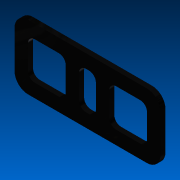
# Autodesk Inventor part: ROV-Side Panel
Saved by Autodesk Inventor 2013 (Build 170138000, 138)
## iProperties
Created: 2014-11-05
Part Number: ROV-Side Panel
Material: Acetal Resin, Black
Document SubType Name: Modeling
Designer: Jeramy
Density: 1 g/cm^3
Author: Jeramy
Autodesk Inventor part; units mm, degrees
ref_plane "YZ Plane" through (0, 0, 0) normal (1, 0, 0) x (0, 1, 0)
ref_plane "XZ Plane" through (0, 0, 0) normal (0, 1, 0) x (-1, 0, 0)
ref_plane "XY Plane" through (0, 0, 0) normal (0, 0, 1) x (1, 0, 0)
sketch "Sketch2" plane through (0, 0, 0) normal (0, 0, 1) x (1, 0, 0)
  line L0 (0, 0) -> (552.641777, 0)
  line L1 (552.641777, 0) -> (552.641777, 244.475)
  line L2 (552.641777, 244.475) -> (0, 244.475)
  line L3 (0, 244.475) -> (0, 0)
  dimension "d6" = 244.475
  constraints: 8 end point, 2 parallel, 1 horizontal, 1 perpendicular
  measures "d6" distance of L1.end L0.end
extrude "Extrusion1" add sketch "Sketch2" along normal blind 19.05
sketch "Sketch3" plane through (0, 0, 19.05) normal (0, 0, 1) x (1, 0, 0)
  line L0 (0, 0) -> (552.641777, 0)
  line L1 (552.641777, 0) -> (552.641777, 244.475)
  line L2 (552.641777, 244.475) -> (0, 244.475)
  line L3 (0, 244.475) -> (0, 0)
  arc A0 (50.896482, 244.475) -> (0, 193.636302) centre (50.799985, 193.675092) ccw
  dimension "d9" = 50.8
  constraints: 2 point on circle, 2 point on line, 1 centre point
  measures "d9" radius of A0
sketch "Sketch3 outline for Extrusion2" plane through (0, 0, 19.05) normal (0, 0, 1) x (1, 0, 0)
  arc A0 (50.896482, 244.475) -> (0, 193.636302) centre (50.799985, 193.675092) ccw
  line L0 (0, 244.475) -> (0, 193.636302)
  line L1 (50.896482, 244.475) -> (0, 244.475)
extrude "Extrusion2" cut sketch "Sketch3 outline for Extrusion2" against normal blind 19.05
sketch "Sketch4" plane through (0, 0, 19.05) normal (0, 0, 1) x (1, 0, 0)
  line L0 (0, 193.713882) -> (0, 0)
  line L1 (0, 0) -> (552.641777, 0)
  line L2 (552.641777, 0) -> (552.641777, 244.475)
  line L3 (552.641777, 244.475) -> (50.703488, 244.475)
  arc A0 (552.641777, 193.713882) -> (500.210663, 244.475) centre (501.841779, 193.701193) ccw
  arc A1 (501.841779, 0) -> (552.641777, 50.788429) centre (501.841778, 50.8) ccw
  arc A2 (0, 50.788429) -> (50.703488, 0) centre (50.799999, 50.799908) ccw
  dimension "d15" = 50.8
  dimension "d16" = 50.8
  dimension "d17" = 50.8
  constraints: 6 point on circle, 6 point on line, 3 centre point
  measures "d15" radius of A0
  measures "d16" radius of A1
  measures "d17" radius of A2
extrude "Extrusion3" cut sketch "Sketch4" against normal blind 19.05 contours A2 L1 L0
sketch "Sketch5" plane through (0, 0, 19.05) normal (0, 0, 1) x (1, 0, 0)
  line L0 (552.641777, 0) -> (552.641777, 244.475)
  line L1 (552.641777, 244.475) -> (50.703488, 244.475)
  arc A0 (552.641777, 193.713882) -> (501.92669, 244.475) centre (501.841792, 193.675071) ccw
  point P0 (0, 0)
  dimension "d20" = 50.8
  constraints: 2 point on circle, 2 point on line, 1 centre point
  measures "d20" radius of A0
extrude "Extrusion4" cut sketch "Sketch5" against normal blind 19.05
sketch "Sketch6" plane through (0, 0, 19.05) normal (0, 0, 1) x (1, 0, 0)
  line L0 (50.703488, 0) -> (552.641777, 0)
  line L1 (552.641777, 0) -> (552.641777, 193.713882)
  arc A0 (501.92669, 0) -> (552.641777, 50.799908) centre (501.841777, 50.799929) ccw
  point P0 (0, 0)
  dimension "d23" = 50.8
  constraints: 2 point on circle, 2 point on line, 1 centre point
  measures "d23" radius of A0
extrude "Extrusion5" cut sketch "Sketch6" against normal blind 19.05
sketch "Sketch7" plane through (0, 0, 19.05) normal (0, 0, 1) x (1, 0, 0)
  arc A0 (552.641777, 193.713882) -> (501.92669, 244.475) centre (501.841792, 193.675071) ccw
  arc A1 (50.703488, 244.475) -> (0, 193.713882) centre (50.799985, 193.675092) ccw
  line L0 (50.799985, 193.675092) -> (193.674985, 193.675092)
  line L1 (193.674985, 193.675092) -> (193.674985, 50.799908)
  line L2 (193.674985, 50.799908) -> (50.799985, 50.799908)
  line L3 (50.799985, 50.799908) -> (50.799985, 193.675092)
  line L4 (501.841792, 193.675071) -> (358.966792, 193.675071)
  line L5 (358.966792, 193.675071) -> (358.966792, 50.799908)
  line L6 (358.966792, 50.799908) -> (501.841792, 50.799908)
  line L7 (501.841792, 50.799908) -> (501.841792, 193.675071)
  point P0 (0, 0)
  dimension "d26" = 142.875
  dimension "d27" = 142.875
  constraints: 16 end point, 4 parallel, 2 horizontal, 2 perpendicular
  measures "d26" distance of L1.end L2.end
  measures "d27" distance of L6.end L5.end
extrude "Extrusion6" cut sketch "Sketch7" against normal blind 19.05 contours L0 L1 L2 L3
sketch "Sketch8" plane through (0, 0, 19.05) normal (0, 0, 1) x (1, 0, 0)
  arc A0 (552.641777, 193.713882) -> (501.92669, 244.475) centre (501.841792, 193.675071) ccw
  line L0 (501.841792, 193.675071) -> (358.966792, 193.675071)
  line L1 (358.966792, 193.675071) -> (358.966792, 50.799908)
  line L2 (358.966792, 50.799908) -> (501.841792, 50.799908)
  line L3 (501.841792, 50.799908) -> (501.841792, 193.675071)
  point P0 (0, 0)
  dimension "d30" = 142.875
  constraints: 8 end point, 2 parallel, 1 horizontal, 1 perpendicular
  measures "d30" distance of L2.end L1.end
extrude "Extrusion7" cut sketch "Sketch8" against normal blind 19.05
sketch "Sketch9" plane through (0, 0, 19.05) normal (0, 0, 1) x (1, 0, 0)
  line L0 (244.474985, 193.675092) -> (308.166792, 193.675092)
  line L1 (308.166792, 193.675092) -> (308.166792, 50.799908)
  line L2 (308.166792, 50.799908) -> (244.474985, 50.799908)
  line L3 (244.474985, 50.799908) -> (244.474985, 193.675092)
  point P0 (193.674985, 193.675092)
  point P1 (0, 0)
  dimension "d33" = 50.8
  constraints: 8 end point, 2 parallel, 1 horizontal, 1 perpendicular
  measures "d33" distance of point (193.675, 193.675) L0.start
extrude "Extrusion8" cut sketch "Sketch9" against normal blind 19.05
fillet "Fillet1" radius 25.4 1 edges at (50.8, 193.6751, 9.525)
fillet "Fillet2" radius 25.4 1 edges at (193.675, 193.6751, 9.525)
fillet "Fillet3" radius 25.4 1 edges at (308.1668, 193.6751, 9.525)
fillet "Fillet4" radius 25.4 1 edges at (501.8418, 193.6751, 9.525)
fillet "Fillet5" radius 25.4 1 edges at (501.8418, 50.7999, 9.525)
fillet "Fillet6" radius 25.4 1 edges at (358.9668, 193.6751, 9.525)
fillet "Fillet7" radius 25.4 1 edges at (358.9668, 50.7999, 9.525)
fillet "Fillet8" radius 25.4 1 edges at (244.475, 50.7999, 9.525)
fillet "Fillet9" radius 25.4 1 edges at (244.475, 193.6751, 9.525)
fillet "Fillet10" radius 25.4 1 edges at (193.675, 50.7999, 9.525)
fillet "Fillet11" radius 25.4 1 edges at (308.1668, 50.7999, 9.525)
fillet "Fillet12" radius 25.4 1 edges at (50.8, 50.7999, 9.525)
body "Solid1"
